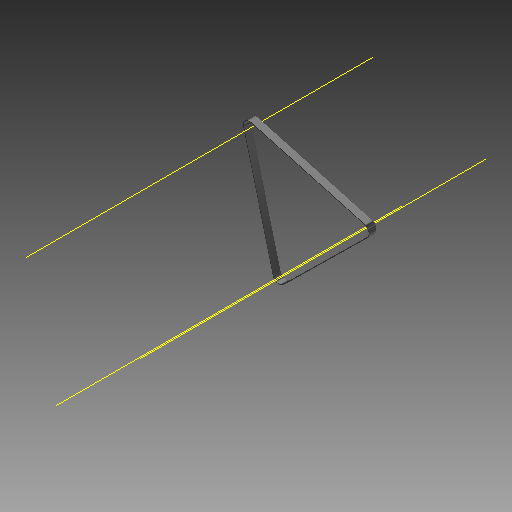
# Autodesk Inventor part: Zahnriemen
Saved by Autodesk Inventor 2018.3 (Build 223284000, 284)
## iProperties
Created: 2018-09-15
Part Number: Zahnriemen
Material: Rubber
Document SubType Name: Modeling
Designer: JochenAlt
Density: 1 g/cm^3
Appearance: Rubber - Black - Version 1.1
CustomPartVersion: 1
Author: JochenAlt
Autodesk Inventor part; units mm, degrees
sketch "Skizzenpfad" plane through (0, 0, 0) normal (0, 0, 1) x (1, 0, 0)
  arc A0 (-110.786, 96.9426) -> (-117.1761, 90.6668) centre (-112.1673, 91.9579) ccw
  arc A1 (-13.0522, 61.811) -> (-15.2986, 70.4828) centre (-16.6799, 65.4981) ccw
  arc A2 (-92.4173, -5.3838) -> (-83.7808, -7.7797) centre (-87.4085, -4.0927) ccw
  line L0 (-92.4173, -5.3838) -> (-117.1761, 90.6668)
  line L1 (-110.786, 96.9426) -> (-15.2986, 70.4828)
  line L2 (-13.0522, 61.811) -> (-83.7808, -7.7797)
  constraints: 6 end point, 6 point on circle, 3 centre point
ref_plane "Querschnittsebene" through (-117.1761, 90.6668, 0) normal (0.2496, -0.9683, 0) x (0, 0, 1)
ref_plane "Arbeitsebene2" through (-112.1673, 91.9579, 0) normal (-1, 0, 0) x (0, 0, 1)
ref_plane "Arbeitsebene3" through (-16.6799, 65.4981, 0) normal (-0.7899, 0.6132, 0) x (0, 0, 1)
ref_plane "Arbeitsebene4" through (-87.4085, -4.0927, 0) normal (0.9218, 0.3878, 0) x (0, 0, 1)
sketch "Querschnitt" plane through (-117.1761, 90.6668, 0) normal (0.2496, -0.9683, 0) x (0, 0, 1)
  line L0 (-3, 0.3) -> (3, 0.3)
  line L1 (3, 0.3) -> (3, -0.3)
  line L2 (3, -0.3) -> (-3, -0.3)
  line L3 (-3, -0.3) -> (-3, 0.3)
  line L4 (-3, 0) -> (3, 0) construction
  point P0 (0, 0)
  point P1 (0, 0)
  dimension "d0" = 6
  dimension "d4" = 0.3
  dimension "d5" = 0.3
  constraints: 10 end point, 3 midpoint, 2 parallel, 1 coincident, 1 horizontal, 1 perpendicular, 1 other
  measures "d0" distance between parallel lines of L1 L3
  measures "d4" distance between parallel lines of L2 L4
  measures "d5" distance between parallel lines of L4 L0
sweep "Riemen" add profiles "Querschnitt" path "Skizzenpfad"
equation "\"d0\" = da_B"
equation "\"d4\" = da_a"
equation "\"d5\" = da_a2"
equation "\"da_B\" = 6"
equation "\"da_pb\" = 2.5"
equation "\"da_a\" = 0.3"
equation "\"da_S\" = 1.5"
equation "\"da_Beta\" = 20deg"
equation "\"da_Ht\" = 0.7"
equation "\"da_H\" = 1.3"
equation "\"da_a2\" = 0.3"
body "Solid1"
